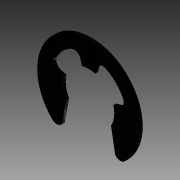
# Autodesk Inventor part: am-0206
Saved by Autodesk Inventor 2014 (Build 180170000, 170)
## iProperties
Category: Drive Base Kit
Company: Autodesk Inc.
Created: 2012-12-19
Part Number: am-0206
Material: Steel
Document SubType Name: Modeling
Designer: Autodesk Inc.
Density: 1 g/cm^3
Catalog Web Link: http://www.andymark.com/product-p/am-0206.htm
Vendor: AndyMark Inc.
Appearance: Black
Author: Autodesk Inc.
Autodesk Inventor part; units mm, degrees
ref_plane "YZ Plane" through (0, 0, 0) normal (1, 0, 0) x (0, 1, 0)
ref_plane "XZ Plane" through (0, 0, 0) normal (0, 1, 0) x (-1, 0, 0)
ref_plane "XY Plane" through (0, 0, 0) normal (0, 0, 1) x (1, 0, 0)
sketch "Sketch1" plane through (0, 0, 0) normal (0, 0, 1) x (1, 0, 0)
  arc A0 (11.7245, -15.68) -> (15.9849, -15.9849) centre (13.9867, -13.9867) ccw
  arc A1 (15.9849, -15.9849) -> (-15.9849, -15.9849) centre (0, 0) ccw
  arc A2 (-15.9849, -15.9849) -> (-11.7245, -15.68) centre (-13.9867, -13.9867) ccw
  line L0 (-11.7245, -15.68) -> (-9.8901, -5.472)
  arc A3 (-10.9218, 2.9106) -> (-9.8901, -5.472) centre (0, 0) ccw
  line L1 (-10.9218, 2.9106) -> (-13.3802, 3.5657)
  arc A4 (-15.1786, 7.5542) -> (-13.3802, 3.5657) centre (-12.6488, 6.2952) ccw
  arc A5 (-7.5542, 15.1786) -> (-15.1786, 7.5542) centre (0, 0) ccw
  arc A6 (-3.5657, 13.3802) -> (-7.5542, 15.1786) centre (-6.2952, 12.6488) ccw
  line L2 (-3.5657, 13.3802) -> (-2.9254, 10.9179)
  arc A7 (2.9254, 10.9179) -> (-2.9254, 10.9179) centre (0, 0) ccw
  line L3 (2.9254, 10.9179) -> (3.5657, 13.3802)
  arc A8 (7.5542, 15.1786) -> (3.5657, 13.3802) centre (6.2952, 12.6488) ccw
  arc A9 (15.1786, 7.5542) -> (7.5542, 15.1786) centre (0, 0) ccw
  arc A10 (13.3802, 3.5657) -> (15.1786, 7.5542) centre (12.6488, 6.2952) ccw
  line L4 (13.3802, 3.5657) -> (10.9218, 2.9106)
  arc A11 (9.8901, -5.472) -> (10.9218, 2.9106) centre (0, 0) ccw
  line L5 (9.8901, -5.472) -> (11.7245, -15.68)
  dimension "d0" = 22.606
  dimension "d2" = 11.303
  constraints: 24 point on circle, 12 centre point, 12 end point
  measures "d0" radius of A1
  measures "d2" radius of A7
extrude "Extrusion1" add sketch "Sketch1" against normal blind 1.27
body "Solid1"
